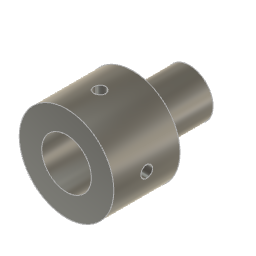
pedal mount v4 (Autodesk Fusion 360 design; units mm, degrees)
Autodesk Fusion 360 part; units mm, degrees
note: some values were not read from the file. Set by a fixed rule: which sketch regions a step uses; which face or edge a step refers to.
sketch "Sketch1" plane through (0, 0, 0) normal (0, 1, 0) x (1, 0, 0)
  circle A0 centre (0, 0) radius 3
  circle A1 centre (0, 0) radius 5
  line L0 (-0.0103, -3) -> (0.0002, 1.55)
  line L1 (3.1387, 1.55) -> (-2.5686, 1.55)
  dimension "d1" = 6
  dimension "d3" = 10
  dimension "d4" = 4.55
  constraint coincident A0.centre A1.centre
  constraint coincident A0 L0.start
  constraint horizontal L1
  constraint coincident A0 L1.end
  measures "d1" diameter of A0
  measures "d3" diameter of A1
  measures "d4" distance of L0.start L0.end
extrude "Extrude1" add sketch "Sketch1" along normal blind 12 contours A0 L1 | A1
move_face "OffsetFaces1" offset -0.25 1 faces at (-1.4888, 8, 2.6045)
sketch "Sketch2" plane through (0, 0, -1.55) normal (0, 0, 1) x (-1, 0, 0)
  line L0 (2.8566, 0) -> (-2.8566, 0)
  line L1 (-2.8566, 0) -> (-2.8566, -12)
  line L2 (-2.8566, -12) -> (2.8566, -12)
  line L3 (2.8566, -12) -> (2.8566, 0)
  circle A0 centre (0, -5.9382) radius 1.1124
extrude "Extrude2" cut sketch "Sketch2" along normal blind 1.5 and the other way blind 6.5 contours A0
sketch "Sketch3" plane through (0, 0, 0) normal (0, -1, 0) x (1, 0, 0)
  arc A0 (2.8566, -1.55) -> (-2.8566, -1.55) centre (0, 0) ccw
  line L0 (2.8566, -1.55) -> (-2.8566, -1.55)
  circle A1 centre (0, 0) radius 5
  circle A2 centre (0, 0) radius 10
  circle A3 centre (0, 0) radius 5.5
  dimension "d12" = 20
  dimension "d13" = 11
  constraint coincident A0.centre A1.centre
  measures "d12" diameter of A2
  measures "d13" diameter of A3
extrude "Extrude3" add sketch "Sketch3" along normal blind 3 contours A0 L0 | A1 | A2 | A3
extrude "Extrude4" add 1 faces at (8.2775, 0, -0.7452) along direction (0, -1, 0) blind 7
fillet "Fillet1" radius 3 1 edges at (-4.6616, 0, 1.8081)
move_face "OffsetFaces2" offset -0.25 1 faces at (4.9752, -4.3333, 0.4978)
extrude "Extrude5" add 1 faces at (8.3599, -7, -0.7576) along direction (0, -1, 0) blind 7
sketch "Sketch4" plane through (0, 0, 0) normal (0, 0, 1) x (1, 0, 0)
  line L0 (0, 0) -> (0, -14.011)
  circle A0 centre (0, -7.0055) radius 1.25
  dimension "d23" = 2.5
  constraint coincident L0.start origin
  constraint vertical L0
  constraint midpoint L0 A0.centre
  measures "d23" diameter of A0
extrude "Extrude6" cut sketch "Sketch4" along normal mid plane 30
sketch "Sketch5" plane through (0, 0, 0) normal (1, 0, 0) x (0, 1, 0)
  line L0 (0, 0) -> (-14.0563, 0)
  circle A0 centre (-7.0282, 0) radius 1.25
  dimension "d26" = 2.5
  constraint coincident L0.start origin
  constraint horizontal L0
  constraint midpoint L0 A0.centre
  measures "d26" diameter of A0
extrude "Extrude7" cut sketch "Sketch5" along normal mid plane 30
